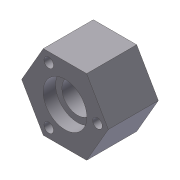
# Autodesk Inventor part: BearingBlock
Saved by Autodesk Inventor 2012 (Build 160160000, 160)
## iProperties
Created: 2012-11-16
Part Number: BearingBlock
Material: Aluminum-6061
Document SubType Name: Modeling
Designer: JesseK
Density: 2.71 g/cm^3
Mass: 62.5118 g
Surface Area: 80.4625 cm^2
Volume: 23.0671 cm^3
Author: JesseK
Autodesk Inventor part; units mm, degrees
ref_plane "YZ Plane" through (0, 0, 0) normal (1, 0, 0) x (0, 1, 0)
ref_plane "XZ Plane" through (0, 0, 0) normal (0, 1, 0) x (-1, 0, 0)
ref_plane "XY Plane" through (0, 0, 0) normal (0, 0, 1) x (1, 0, 0)
sketch "Sketch1" plane through (0, 0, 0) normal (0, 0, 1) x (1, 0, 0)
  line L0 (21.997, 0) -> (10.9985, -19.05)
  line L1 (10.9985, -19.05) -> (-10.9985, -19.05)
  line L2 (-10.9985, -19.05) -> (-21.997, 0)
  line L3 (-21.997, 0) -> (-10.9985, 19.05)
  line L4 (-10.9985, 19.05) -> (10.9985, 19.05)
  line L5 (10.9985, 19.05) -> (21.997, 0)
  circle A0 centre (0, 0) radius 7.9375
  line L6 (8.2489, 14.2875) -> (16.4978, 0) construction
  line L7 (16.4978, 0) -> (8.2489, -14.2875) construction
  line L8 (8.2489, -14.2875) -> (-8.2489, -14.2875) construction
  line L9 (-8.2489, -14.2875) -> (-16.4978, 0) construction
  line L10 (-16.4978, 0) -> (-8.2489, 14.2875) construction
  line L11 (-8.2489, 14.2875) -> (8.2489, 14.2875) construction
  circle A1 centre (-8.2489, 14.2875) radius 2.4384
  circle A2 centre (16.4978, 0) radius 2.4384
  circle A3 centre (-8.2489, -14.2875) radius 2.4384
  dimension "d0" = 15.875
  dimension "d1" = 38.1
  dimension "d2" = 28.575
  dimension "d3" = 4.8768
  constraints: 24 end point, 6 coincident, 4 centre point, 2 equal radius, 1 horizontal, 26 other
  measures "d0" diameter of A0
  measures "d1" distance between parallel lines of L1 L4
  measures "d2" distance between parallel lines of L8 L11
  measures "d3" diameter of A1
extrude "Extrusion1" add sketch "Sketch1" along normal blind 25.4
sketch "Sketch2" plane through (0, 0, 25.4) normal (0, 0, 1) x (1, 0, 0)
  circle A0 centre (0, 0) radius 7.9375 projected
  circle A1 centre (0, 0) radius 11.1125
  dimension "d6" = 22.225
  constraints: 1 centre point, 1 coincident
  measures "d6" diameter of A1
extrude "Extrusion2" cut sketch "Sketch2" against normal blind 6.35
sketch "Sketch3" plane through (0, 0, 0) normal (0, 0, -1) x (-1, 0, 0)
  circle A0 centre (0, 0) radius 7.9375 projected
  circle A1 centre (0, 0) radius 11.1125
  dimension "d9" = 22.225
  constraints: 1 centre point, 1 coincident
  measures "d9" diameter of A1
extrude "Extrusion3" cut sketch "Sketch3" against normal blind 6.35
body "Solid1"
